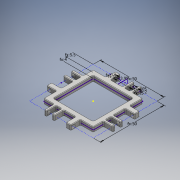
# Autodesk Inventor part: square
Saved by Autodesk Inventor 2016 (Build 200138000, 138)
## iProperties
Created: 2016-11-12
Part Number: square
Material: Generic
Document SubType Name: Modeling
Designer: Chris
Density: 1 g/cm^3
Appearance: Default
Author: Chris
Autodesk Inventor part; units mm, degrees
ref_plane "XZ Plane" through (0, 0, 0) normal (0, 1, 0) x (-1, 0, 0)
ref_plane "XY Plane" through (0, 0, 0) normal (0, 0, 1) x (1, 0, 0)
sketch "Sketch1" plane through (0, 0, 0) normal (0, 0, 1) x (1, 0, 0)
  line L0 (-25, -25) -> (25, -25) construction
  line L1 (25, -25) -> (25, 25) construction
  line L2 (25, 25) -> (-25, 25) construction
  line L3 (-25, 25) -> (-25, -25) construction
  line L4 (-19.5, 19.5) -> (19.5, 19.5)
  line L5 (19.5, 19.5) -> (19.5, -19.5)
  line L6 (19.5, -19.5) -> (-19.5, -19.5)
  line L7 (-19.5, -19.5) -> (-19.5, 19.5)
  line L8 (15.5, 15.5) -> (-15.5, 15.5)
  line L9 (-15.5, 15.5) -> (-15.5, -15.5)
  line L10 (-15.5, -15.5) -> (15.5, -15.5)
  line L11 (15.5, -15.5) -> (15.5, 15.5)
  line L12 (-7.5, 25) -> (7.5, 25) construction
  line L13 (-9.475, 25) -> (-5.525, 25) construction
  line L14 (5.475, 25) -> (9.525, 25) construction
  line L15 (5.475, 25) -> (3.475, 25) construction
  line L16 (9.525, 25) -> (11.525, 25) construction
  point P0 (0, 0)
  point P1 (-25, 0)
  point P2 (0, 25)
  point P3 (-7.5, 25)
  point P4 (7.5, 25)
  dimension "d2" = 50
  dimension "d3" = 50
  dimension "d4" = 5.5
  dimension "d5" = 4
  dimension "d6" = 15
  dimension "d9" = 3.95
  dimension "d10" = 4.05
  dimension "d11" = 2
  constraints: 34 end point, 8 coincident, 6 horizontal, 6 parallel, 5 midpoint, 3 perpendicular, 1 collinear, 1 horizontal alignment, 1 vertical alignment, 6 other
  measures "d2" distance of L2.end L1.end
  measures "d3" distance of L1.end L0.end
  measures "d4" distance between parallel lines of L4 L2
  measures "d5" distance between parallel lines of L8 L4
  measures "d6" distance of L12.start L12.end
  measures "d9" distance of L13.start L13.end
  measures "d10" distance of L14.start L14.end
  measures "d11" distance of L14.end L16.end
extrude "Extrusion1" add sketch "Sketch1" along normal mid plane 4
ref_plane "Work Plane1" through (-9.475, 25, 0) normal (1, 0, 0) x (0, 1, 0)
ref_plane "Work Plane2" through (-5.525, 25, 0) normal (1, 0, 0) x (0, 1, 0)
ref_plane "Work Plane3" through (3.475, 25, 0) normal (1, 0, 0) x (0, 1, 0)
ref_plane "Work Plane4" through (5.475, 25, 0) normal (1, 0, 0) x (0, 1, 0)
ref_plane "Work Plane5" through (9.525, 25, 0) normal (1, 0, 0) x (0, 1, 0)
ref_plane "Work Plane6" through (11.525, 25, 0) normal (1, 0, 0) x (0, 1, 0)
sketch "Sketch2" plane through (0, 0, 0) normal (1, 0, 0) x (0, 1, 0)
  line L0 (19.5, -2) -> (19.5, 2) projected
  line L1 (19.5, 2) -> (19.5, -2) projected
  line L2 (19.5, 2) -> (27, 2)
  line L3 (27, 2) -> (27, -2)
  line L4 (27, -2) -> (19.5, -2)
  line L5 (19.5, -2) -> (19.5, 2)
  circle A0 centre (25, 0) radius 2 construction
  point P0 (0, 0)
  constraints: 8 end point, 2 parallel, 2 tangent, 1 centre point, 1 coincident, 1 horizontal, 1 perpendicular
extrude "Extrusion2" add sketch "Sketch2" against normal up to surface (3.95 mm away) from surface at -5.525
extrude "Extrusion3" add sketch "Sketch2" along normal up to surface (2 mm away) from surface at 3.475
extrude "Extrusion4" add sketch "Sketch2" along normal up to surface (2 mm away) from surface at 9.525
sketch "Sketch3" plane through (0, 0, 0) normal (0, 0, 1) x (1, 0, 0)
  line L0 (25, 25) -> (-25, 25) construction
  line L1 (-9.475, 25) -> (-8.975, 25)
  line L2 (-9.475, 26.5) -> (-9.475, 25)
  line L3 (-5.525, 25) -> (-6.025, 25)
  line L4 (-5.525, 25) -> (-5.525, 26.5)
  line L5 (5.475, 25) -> (5.975, 25)
  line L6 (5.475, 25) -> (5.475, 26.5)
  line L7 (9.525, 25) -> (9.525, 26.5)
  line L8 (9.525, 25) -> (9.025, 25)
  arc A0 (-5.525, 26.5) -> (-6.025, 25) centre (-3.525, 25) ccw
  arc A1 (-8.975, 25) -> (-9.475, 26.5) centre (-11.475, 25) ccw
  arc A2 (5.975, 25) -> (5.475, 26.5) centre (3.475, 25) ccw
  arc A3 (9.525, 26.5) -> (9.025, 25) centre (11.525, 25) ccw
  point P0 (0, 0)
  dimension "d18" = 3
  dimension "d31" = 0.5
  constraints: 16 end point, 8 point on circle, 4 centre point, 4 equal length, 4 vertical, 3 equal radius, 2 horizontal, 1 point on line, 7 other
  measures "d18" diameter of L2.start L1
  measures "d31" distance of L1.start L1.end
revolve "Revolution1" cut sketch "Sketch3" angle 360 about axis through (25, 25, 0) along (-1, 0, 0) contours L2 A1 L1 | L3 A0 L4
revolve "Revolution2" add sketch "Sketch3" angle 360 about axis through (25, 25, 0) along (-1, 0, 0) contours L6 A2 L5 | L8 A3 L7
pattern_circular "Circular Pattern1" count 4 over 360 about axis through (0, 0, -10) along (0, 0, 1) of "Extrusion2", "Extrusion3", "Extrusion4", "Revolution2", "Revolution1"
fillet "Fillet2" radius 1 8 edges at (-19.5, 19.5, 0) (-15.5, 15.5, 0) (15.5, 15.5, 0) (19.5, 19.5, 0) (15.5, -15.5, 0) (19.5, -19.5, 0) (-15.5, -15.5, 0) (-19.5, -19.5, 0)
fillet "Fillet3" radius 0.75 48 edges at (-9.475, 19.5, 0) (-5.525, 19.5, 0) (3.475, 19.5, 0) (5.475, 19.5, 0) (9.525, 19.5, 0) (11.525, 19.5, 0) (19.5, 9.475, 0) (19.5, 5.525, 0) (19.5, -3.475, 0) (19.5, -5.475, 0) (19.5, -9.525, 0) (19.5, -11.525, 0) (9.475, -19.5, 0) (5.525, -19.5, 0) (-3.475, -19.5, 0) (-5.475, -19.5, 0) (-9.525, -19.5, 0) (-11.525, -19.5, 0) (-19.5, -9.475, 0) (-19.5, -5.525, 0) (-19.5, 3.475, 0) (-19.5, 5.475, 0) (-19.5, 9.525, 0) (-19.5, 11.525, 0) (-27, 11.525, 0) (-27, 9.525, 0) (-27, 5.475, 0) (-27, 3.475, 0) (-27, -5.525, 0) (-27, -9.475, 0) (-11.525, -27, 0) (-9.525, -27, 0) (-5.475, -27, 0) (-3.475, -27, 0) (5.525, -27, 0) (9.475, -27, 0) (27, -11.525, 0) (27, -9.525, 0) (27, -5.475, 0) (27, -3.475, 0) (27, 9.475, 0) (27, 5.525, 0) (11.525, 27, 0) (9.525, 27, 0) (5.475, 27, 0) (3.475, 27, 0) (-5.525, 27, 0) (-9.475, 27, 0)
chamfer "Chamfer1" distance 0.4 angle 45 208 edges at (0, 15.5, 2) (15.2071, 15.2071, 2) (15.5, 0, 2) (15.2071, -15.2071, 2) (0, -15.5, 2) (-15.2071, -15.2071, 2) (-15.5, 0, 2) (-15.2071, 15.2071, 2) (-19.5, 15.3875, -2) (-19.2071, 19.2071, -2) (-14.3625, 19.5, -2) (-9.6947, 19.7197, -2) (-9.475, 23.25, -2) (-9.2553, 26.7803, -2) (-7.5, 27, -2) (-5.7447, 26.7803, -2) (-5.525, 23.25, -2) (-5.3053, 19.7197, -2) (-1.025, 19.5, -2) (3.2553, 19.7197, -2) (3.475, 23.25, -2) (3.6947, 26.7803, -2) (4.475, 27, -2) (5.2553, 26.7803, -2) (5.475, 23.25, -2) (5.6947, 19.7197, -2) (7.5, 19.5, -2) (9.3053, 19.7197, -2) (9.525, 23.25, -2) (9.7447, 26.7803, -2) (10.525, 27, -2) (11.3053, 26.7803, -2) (11.525, 23.25, -2) (11.7447, 19.7197, -2) (15.3875, 19.5, -2) (19.2071, 19.2071, -2) (19.5, 14.3625, -2) (19.7197, 9.6947, -2) (23.25, 9.475, -2) (26.7803, 9.2553, -2) (27, 7.5, -2) (26.7803, 5.7447, -2) (23.25, 5.525, -2) (19.7197, 5.3053, -2) (19.5, 1.025, -2) (19.7197, -3.2553, -2) (23.25, -3.475, -2) (26.7803, -3.6947, -2) (27, -4.475, -2) (26.7803, -5.2553, -2) (23.25, -5.475, -2) (19.7197, -5.6947, -2) (19.5, -7.5, -2) (19.7197, -9.3053, -2) (23.25, -9.525, -2) (26.7803, -9.7447, -2) (27, -10.525, -2) (26.7803, -11.3053, -2) (23.25, -11.525, -2) (19.7197, -11.7447, -2) (19.5, -15.3875, -2) (19.2071, -19.2071, -2) (14.3625, -19.5, -2) (9.6947, -19.7197, -2) (9.475, -23.25, -2) (9.2553, -26.7803, -2) (7.5, -27, -2) (5.7447, -26.7803, -2) (5.525, -23.25, -2) (5.3053, -19.7197, -2) (1.025, -19.5, -2) (-3.2553, -19.7197, -2) (-3.475, -23.25, -2) (-3.6947, -26.7803, -2) (-4.475, -27, -2) (-5.2553, -26.7803, -2) (-5.475, -23.25, -2) (-5.6947, -19.7197, -2) (-7.5, -19.5, -2) (-9.3053, -19.7197, -2) (-9.525, -23.25, -2) (-9.7447, -26.7803, -2) (-10.525, -27, -2) (-11.3053, -26.7803, -2) (-11.525, -23.25, -2) (-11.7447, -19.7197, -2) (-15.3875, -19.5, -2) (-19.2071, -19.2071, -2) (-19.5, -14.3625, -2) (-19.7197, -9.6947, -2) (-23.25, -9.475, -2) (-26.7803, -9.2553, -2) (-27, -7.5, -2) (-26.7803, -5.7447, -2) (-23.25, -5.525, -2) (-19.7197, -5.3053, -2) (-19.5, -1.025, -2) (-19.7197, 3.2553, -2) (-23.25, 3.475, -2) (-26.7803, 3.6947, -2) (-27, 4.475, -2) (-26.7803, 5.2553, -2) (-23.25, 5.475, -2) (-19.7197, 5.6947, -2) (-19.5, 7.5, -2) (-19.7197, 9.3053, -2) (-23.25, 9.525, -2) (-26.7803, 9.7447, -2) (-19.5, 7.5, 2) (-19.7197, 5.6947, 2) (-23.25, 5.475, 2) (-26.7803, 5.2553, 2) (-27, 4.475, 2) (-26.7803, 3.6947, 2) (-23.25, 3.475, 2) (-19.7197, 3.2553, 2) (-19.5, -1.025, 2) (-19.7197, -5.3053, 2) (-23.25, -5.525, 2) (-26.7803, -5.7447, 2) (-27, -7.5, 2) (-26.7803, -9.2553, 2) (-23.25, -9.475, 2) (-19.7197, -9.6947, 2) (-19.5, -14.3625, 2) (-19.2071, -19.2071, 2) (-15.3875, -19.5, 2) (-11.7447, -19.7197, 2) (-11.525, -23.25, 2) (-11.3053, -26.7803, 2) (-10.525, -27, 2) (-9.7447, -26.7803, 2) (-9.525, -23.25, 2) (-9.3053, -19.7197, 2) (-7.5, -19.5, 2) (-5.6947, -19.7197, 2) (-5.475, -23.25, 2) (-5.2553, -26.7803, 2) (-4.475, -27, 2) (-3.6947, -26.7803, 2) (-3.475, -23.25, 2) (-3.2553, -19.7197, 2) (1.025, -19.5, 2) (5.3053, -19.7197, 2) (5.525, -23.25, 2) (5.7447, -26.7803, 2) (7.5, -27, 2) (9.2553, -26.7803, 2) (9.475, -23.25, 2) (9.6947, -19.7197, 2) (14.3625, -19.5, 2) (19.2071, -19.2071, 2) (19.5, -15.3875, 2) (19.7197, -11.7447, 2) (23.25, -11.525, 2) (26.7803, -11.3053, 2) (27, -10.525, 2) (26.7803, -9.7447, 2) (23.25, -9.525, 2) (19.7197, -9.3053, 2) (19.5, -7.5, 2) (19.7197, -5.6947, 2) (23.25, -5.475, 2) (26.7803, -5.2553, 2) (27, -4.475, 2) (26.7803, -3.6947, 2) (23.25, -3.475, 2) (19.7197, -3.2553, 2) (19.5, 1.025, 2) (19.7197, 5.3053, 2) (23.25, 5.525, 2) (26.7803, 5.7447, 2) (27, 7.5, 2) (26.7803, 9.2553, 2) (23.25, 9.475, 2) (19.7197, 9.6947, 2) (19.5, 14.3625, 2) (19.2071, 19.2071, 2) (15.3875, 19.5, 2) (11.7447, 19.7197, 2) (11.525, 23.25, 2) (11.3053, 26.7803, 2) (10.525, 27, 2) (9.7447, 26.7803, 2) (9.525, 23.25, 2) (9.3053, 19.7197, 2) (7.5, 19.5, 2) (5.6947, 19.7197, 2) (5.475, 23.25, 2) (5.2553, 26.7803, 2) (4.475, 27, 2) (3.6947, 26.7803, 2) (3.475, 23.25, 2) (3.2553, 19.7197, 2) (-1.025, 19.5, 2) (-5.3053, 19.7197, 2) (-5.525, 23.25, 2) (-5.7447, 26.7803, 2) (-7.5, 27, 2) (-9.2553, 26.7803, 2) (-9.475, 23.25, 2) (-9.6947, 19.7197, 2) (-14.3625, 19.5, 2) (-19.2071, 19.2071, 2) (-19.5, 15.3875, 2) (-19.7197, 11.7447, 2) (-23.25, 11.525, 2) (-26.7803, 11.3053, 2)
equation "\"d2\" = sidelength"
equation "\"d3\" = sidelength"
equation "\"d4\" = springlength"
equation "\"d5\" = diam"
equation "\"d6\" = matespace"
equation "\"d9\" = fingerwidth - 0.5 * tolerance"
equation "\"d10\" = fingerwidth + 0.5 * tolerance"
equation "\"d11\" = springwidth"
equation "\"d7\" = diam"
equation "\"d12\" = diam"
equation "\"d14\" = diam"
equation "\"d16\" = diam"
equation "\"d18\" = dentdiam"
equation "\"sidelength\" = 50"
equation "\"diam\" = 4"
equation "\"dent\" = 0.5"
equation "\"dentdiam\" = 3"
equation "\"tolerance\" = 0.1"
equation "\"fingerwidth\" = 4"
equation "\"springwidth\" = 2"
equation "\"matespace\" = 15"
equation "\"springlength\" = 5.5"
body "Solid1"
